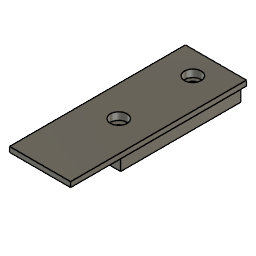
Laser Mount (Autodesk Fusion 360 design; units mm, degrees)
part number: 2026-06-20-05-23-10-439
Autodesk Fusion 360 part; units mm, degrees
sketch "Sketch1" plane through (0, 0, 0) normal (0, 0, 1) x (1, 0, 0)
  line L0 (-30.5, 32.5) -> (30.5, 32.5)
  line L1 (32.5, 30.5) -> (32.5, -30.5)
  line L2 (30.5, -32.5) -> (-30.5, -32.5)
  line L3 (-32.5, -30.5) -> (-32.5, 30.5)
  line L4 (-32.5, 32.5) -> (32.5, -32.5) construction
  line L5 (32.5, 32.5) -> (-32.5, -32.5) construction
  circle A0 centre (0, 0) radius 2.5
  circle A1 centre (0, 10) radius 2.5
  circle A2 centre (0, 20) radius 3.5
  circle A3 centre (0, -10) radius 2.5
  circle A4 centre (0, -20) radius 2.5
  circle A5 centre (10, -20) radius 2.5
  circle A6 centre (10, 0) radius 2.5
  circle A7 centre (10, 20) radius 2.5
  circle A8 centre (20, -20) radius 2.5
  circle A9 centre (20, 20) radius 2.5
  line L6 (17.5, 10) -> (17.5, -10)
  line L7 (22.5, -10) -> (22.5, 10)
  arc A10 (22.5, 10) -> (17.5, 10) centre (20, 10) ccw
  arc A11 (17.5, -10) -> (22.5, -10) centre (20, -10) ccw
  line L8 (29, 3) -> (29, -3)
  line L9 (26, -3) -> (26, 3)
  arc A12 (29, 3) -> (26, 3) centre (27.5, 3) ccw
  arc A13 (26, -3) -> (29, -3) centre (27.5, -3) ccw
  arc A14 (29, 23) -> (26, 23) centre (27.5, 23) ccw
  line L10 (29, 23) -> (29, 17)
  arc A15 (26, 17) -> (29, 17) centre (27.5, 17) ccw
  line L11 (26, 17) -> (26, 23)
  arc A16 (26, -23) -> (29, -23) centre (27.5, -23) ccw
  line L12 (29, -17) -> (29, -23)
  line L13 (26, -23) -> (26, -17)
  arc A17 (29, -17) -> (26, -17) centre (27.5, -17) ccw
  circle A18 centre (-10, -20) radius 2.5
  line L14 (-26, -3) -> (-26, 3)
  line L15 (-26, 17) -> (-26, 23)
  arc A19 (-29, -3) -> (-26, -3) centre (-27.5, -3) ccw
  circle A20 centre (-10, 20) radius 2.5
  circle A21 centre (-20, -20) radius 2.5
  line L16 (-29, 23) -> (-29, 17)
  circle A22 centre (-20, 20) radius 2.5
  arc A23 (-17.5, 10) -> (-22.5, 10) centre (-20, 10) ccw
  arc A24 (-26, 23) -> (-29, 23) centre (-27.5, 23) ccw
  arc A25 (-22.5, -10) -> (-17.5, -10) centre (-20, -10) ccw
  arc A26 (-26, 3) -> (-29, 3) centre (-27.5, 3) ccw
  line L17 (-17.5, 10) -> (-17.5, -10)
  line L18 (-29, 3) -> (-29, -3)
  circle A27 centre (-10, 0) radius 2.5
  arc A28 (-29, -23) -> (-26, -23) centre (-27.5, -23) ccw
  line L19 (-22.5, -10) -> (-22.5, 10)
  line L20 (-26, -23) -> (-26, -17)
  arc A29 (-26, -17) -> (-29, -17) centre (-27.5, -17) ccw
  arc A30 (-29, 17) -> (-26, 17) centre (-27.5, 17) ccw
  line L21 (-29, -17) -> (-29, -23)
  arc A31 (-30.5, 32.5) -> (-32.5, 30.5) centre (-30.5, 30.5) ccw
  arc A32 (32.5, 30.5) -> (30.5, 32.5) centre (30.5, 30.5) ccw
  arc A33 (30.5, -32.5) -> (32.5, -30.5) centre (30.5, -30.5) ccw
  arc A34 (-32.5, -30.5) -> (-30.5, -32.5) centre (-30.5, -30.5) ccw
  circle A35 centre (0, 20) radius 1.65
  circle A36 centre (0, 20) radius 3.35
  circle A37 centre (0, -20) radius 1.65
  circle A38 centre (0, -20) radius 2.35
  dimension "d1" = 65
  dimension "d2" = 65
  dimension "d3" = 5
  dimension "d8" = 7
  dimension "d11" = 0
  dimension "d12" = -10
  dimension "d13" = 5
  dimension "d14" = 5
  dimension "d16" = 5
  dimension "d17" = 3
  dimension "d19" = 3
  dimension "d20" = 3
  dimension "d21" = 3
  dimension "d22" = 3
  dimension "d23" = 3
  dimension "d24" = 2
  dimension "d25" = 2
  dimension "d26" = 2
  dimension "d27" = 2
  dimension "d42" = 3.3
  dimension "d43" = 6.7
  dimension "d44" = 3.3
  dimension "d45" = 4.7
  constraint horizontal L0
  constraint perpendicular L0 L1
  constraint parallel L0 L2
  constraint parallel L1 L3
  constraint coincident L4 A0.centre
  constraint coincident L5 A0.centre
  constraint coincident A0.centre origin
  constraint tangent L6 A10
  constraint tangent L6 A11
  constraint vertical L6
  constraint tangent L7 A11
  constraint tangent L7 A10
  constraint parallel L6 L7
  constraint tangent L8 A13
  constraint parallel L1 L8
  constraint tangent L9 A12
  constraint parallel L8 L9
  constraint tangent L10 A15
  constraint tangent A14 L11
  constraint parallel L10 L11
  constraint tangent A16 L12
  constraint tangent L13 A17
  constraint parallel L12 L13
  constraint coincident L4.start L3
  constraint coincident L4.start L0
  constraint tangent L3 A31
  constraint tangent L0 A31
  constraint coincident L5.start L0
  constraint coincident L5.start L1
  constraint tangent L0 A32
  constraint tangent L1 A32
  constraint coincident L4.end L1
  constraint coincident L4.end L2
  constraint tangent L1 A33
  constraint tangent L2 A33
  constraint coincident L5.end L2
  constraint coincident L5.end L3
  constraint tangent L2 A34
  constraint tangent L3 A34
  constraint concentric A2 A35
  constraint concentric A2 A36
  constraint concentric A4 A37
  constraint concentric A37 A38
  measures "d1" distance of L4.end L5.end
  measures "d2" distance of L5.start L4.end
  measures "d3" diameter of A0
  measures "d8" diameter of A2
  measures "d13" diameter of A6
  measures "d14" diameter of A7
  measures "d16" diameter of A9
  measures "d17" diameter of A13
  measures "d19" diameter of A12
  measures "d20" diameter of A15
  measures "d21" diameter of A14
  measures "d22" diameter of A16
  measures "d23" diameter of A17
  measures "d24" radius of A31
  measures "d25" radius of A32
  measures "d26" radius of A33
  measures "d27" radius of A34
  measures "d42" diameter of A35
  measures "d43" diameter of A36
  measures "d44" diameter of A37
  measures "d45" diameter of A38
ref_plane "WorkPlane1" through (0, 0, 3) normal (0, 0, 1) x (1, 0, 0)
sketch "Sketch3" plane through (0, 0, 3) normal (0, 0, 1) x (1, 0, 0)
  line L0 (13.5, 32.5) -> (-13.5, 32.5)
  line L1 (-13.5, 32.5) -> (-13.5, -32.5)
  line L2 (-13.5, -32.5) -> (13.5, -32.5)
  line L3 (13.5, -32.5) -> (13.5, 32.5)
  line L4 (13.5, 32.5) -> (-13.5, -32.5) construction
  line L5 (-13.5, 32.5) -> (13.5, -32.5) construction
  circle A0 centre (0, 20) radius 3.35
  circle A1 centre (0, -20) radius 2.35
  circle A2 centre (0, 20) radius 2.15
  circle A3 centre (0, -20) radius 1.65
  dimension "d33" = 27
  dimension "d34" = 65
  dimension "d67" = 6.7
  dimension "d68" = 4.7
  dimension "d69" = 4.3
  dimension "d70" = 3.3
  constraint horizontal L0
  constraint perpendicular L0 L1
  constraint parallel L0 L2
  constraint parallel L1 L3
  constraint coincident L4 origin
  constraint coincident L5 origin
  constraint concentric A0 A2
  constraint concentric A1 A3
  measures "d33" distance of L1.end L2.end
  measures "d34" distance of L0.end L1.end
  measures "d67" diameter of A0
  measures "d68" diameter of A1
  measures "d69" diameter of A2
  measures "d70" diameter of A3
ref_plane "WorkPlane2" through (0, 0, 12) normal (0, 0, 1) x (1, 0, 0)
sketch "Sketch4" plane through (0, 0, 12) normal (0, 0, 1) x (1, 0, 0)
  line L0 (16.5, 32.5) -> (-16.5, 32.5)
  line L1 (-16.5, 32.5) -> (-16.5, -32.5)
  line L2 (16.5, -32.5) -> (16.5, 32.5)
  line L3 (-16.5, -32.5) -> (-16.5, -62.5)
  line L4 (-16.5, -62.5) -> (16.5, -62.5)
  line L5 (16.5, -62.5) -> (16.5, -32.5)
  circle A0 centre (0, 20) radius 2.15
  circle A1 centre (0, -20) radius 1.65
  dimension "d38" = 30
  dimension "d39" = 33
  constraint parallel L1 L3
  constraint perpendicular L3 L4
  constraint perpendicular L4 L5
  measures "d38" distance of L1.end L3.end
  measures "d39" distance of L3.end L4.end
ref_plane "WorkPlane3" through (0, 0, 14.8) normal (0, 0, 1) x (1, 0, 0)
sketch "Sketch5" plane through (0, 0, 14.8) normal (0, 0, 1) x (1, 0, 0)
  circle A0 centre (0, 20) radius 4.5
  circle A1 centre (0, -20) radius 4.5
  dimension "d61" = 9
  dimension "d62" = 9
  measures "d61" diameter of A0
  measures "d62" diameter of A1
extrude "Extrude8" add sketch "Sketch3" along normal blind 9 contours L0 L1 L2 L3 | A0 | A1 makes body 1
extrude "Extrude9" add sketch "Sketch4" along normal blind 2.8 bodies 1
extrude "Extrude10" cut sketch "Sketch5" against normal blind 4 bodies 1
extrude "Extrude11" add sketch "Sketch3" against normal blind 2 contours A0 bodies 1
fillet "Fillet3" radius 1 1 edges at (-3.1233, 21.2114, 1) on bodies 1
extrude "Extrude12" add sketch "Sketch3" against normal blind 1.5 contours A1 bodies 1
fillet "Fillet4" radius 0.5 1 edges at (-2.191, -19.1502, 1.5) on bodies 1
extrude "Extrude1" add sketch "Sketch1" along normal blind 3 separate body contours L0 L1 L2 L3 A31 A32 A33 A34 makes body 2
hidden bodies 2
equation "d43 = 7 mm - 0.3 mm"
equation "d45 = 5 mm - 0.3 mm"
equation "d67 = 7 mm - 0.3 mm"
equation "d68 = 5 mm - 0.3 mm"
named bodies: "Laser Plate", "Laser Mount"
